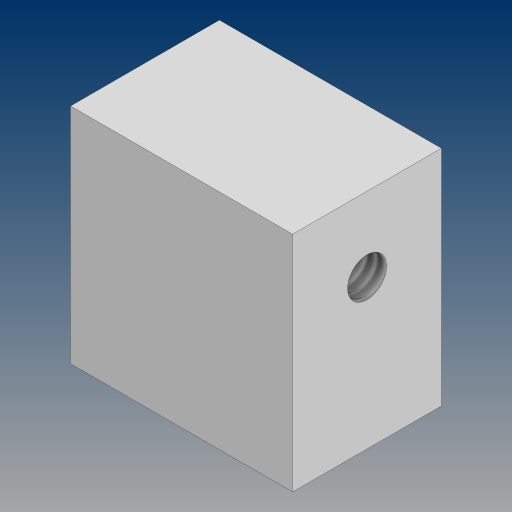
# Autodesk Inventor part: Intake Pivot Billet
Saved by Autodesk Inventor 2024.3 (Build 283343000, 343)
## iProperties
Created: 2024-08-01
Part Number: Intake Pivot Billet
Material: Generic
Document SubType Name: Modeling
Designer: Kenji
Density: 1 g/cm^3
Appearance: Default
Author: Kenji
Autodesk Inventor part; units mm, degrees
ref_plane "YZ Plane" through (0, 0, 0) normal (1, 0, 0) x (0, 1, 0)
ref_plane "XZ Plane" through (0, 0, 0) normal (0, 1, 0) x (-1, 0, 0)
ref_plane "XY Plane" through (0, 0, 0) normal (0, 0, 1) x (1, 0, 0)
sketch "Sketch1" plane through (0, 0, 0) normal (1, 0, 0) x (0, 1, 0)
  circle A0 centre (0, 0) radius 2.3813
  line L0 (9.525, 9.525) -> (-19.05, 9.525)
  line L1 (-19.05, 9.525) -> (-19.05, -9.525)
  line L2 (-19.05, -9.525) -> (9.525, -9.525)
  line L3 (9.525, -9.525) -> (9.525, 9.525)
  dimension "d0" = 4.7625
  dimension "d1" = 19.05
  dimension "d2" = 28.575
  dimension "d3" = 19.05
  dimension "d4" = 9.525
  constraints: 8 end point, 2 parallel, 1 centre point, 1 coincident, 1 horizontal, 1 perpendicular
  measures "d0" diameter of A0
  measures "d1" distance of L1.end L0.end
  measures "d2" distance between parallel lines of L1 L3
  measures "d3" distance from line of L1 A0.centre
  measures "d4" distance from line of L0 A0.centre
extrude "Extrusion1" add sketch "Sketch1" along normal blind 28.4226
sketch "Sketch2" plane through (0, -19.05, -9.525) normal (0, -1, 0) x (1, 0, 0)
  line L0 (0, 19.05) -> (0, 0) projected
  line L1 (0, 0) -> (28.4226, 0) projected
  line L2 (28.4226, 19.05) -> (28.4226, 0) projected
  line L3 (0, 19.05) -> (28.4226, 19.05) projected
  point P0 (0, 9.525)
  point P1 (6.35, 9.525)
  dimension "d7" = 9.525
  dimension "d8" = 6.35
  measures "d7" distance from line of L3 point (6.35, 9.525)
  measures "d8" distance from line of L0 point (6.35, 9.525)
hole "Hole1" at (6.35, -19.05, 0) direction (0, 1, 0) diameter 4.9784 depth 15.24 thread size "1/4-20 UNC" class "2B" standard "ANSI Unified Screw Threads"
sketch "Sketch3" plane through (0, 0, 0) normal (-1, 0, 0) x (0, 0, 1)
  point P0 (0, 0)
  point P1 (0, 0)
  constraints: 1 coincident
hole "Hole2" at (0, 0, 0) direction (1, 0, 0) diameter 4.9784 depth 28.4226 thread size "1/4-20 UNC" class "2B" standard "ANSI Unified Screw Threads"
body "Solid1"
